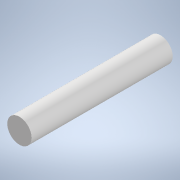
# Autodesk Inventor part: Marcador
Saved by Autodesk Inventor 2021 (Build 250183000, 183)
## iProperties
Created: 2022-10-25
Part Number: Marcador
Material: Generic
Document SubType Name: Modeling
Designer: zulet
Mass: 24.4377 g
Surface Area: 60.6681 cm^2
Volume: 24.4377 cm^3
Density: 1 g/cm^3
Appearance: Default
Author: zulet
Autodesk Inventor part; units mm, degrees
ref_plane "YZ Plane" through (0, 0, 0) normal (1, 0, 0) x (0, 1, 0)
ref_plane "XZ Plane" through (0, 0, 0) normal (0, 1, 0) x (-1, 0, 0)
ref_plane "XY Plane" through (0, 0, 0) normal (0, 0, 1) x (1, 0, 0)
sketch "Sketch1" plane through (0, 0, 0) normal (0, 0, 1) x (1, 0, 0)
  circle A0 centre (0, -89.625) radius 8.75 projected
  point P0 (0, 0)
  dimension "d0" = 101.6
extrude "Extrusion1" add sketch "Sketch1" along normal mid plane 101.6
body "Solid1"
